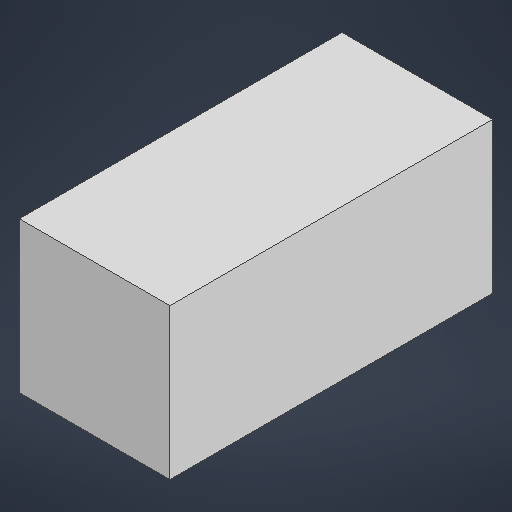
# Autodesk Inventor part: shootingstand
Saved by Autodesk Inventor 2026.2 (Build 302298000, 298)
## iProperties
Created: 2026-03-08
Part Number: shootingstand
Material: Generic
Document SubType Name: Modeling
Designer: danda
Density: 1 g/cm^3
Appearance: Default
Author: danda
Autodesk Inventor part; units mm, degrees
ref_plane "YZ Plane" through (0, 0, 0) normal (1, 0, 0) x (0, 1, 0)
ref_plane "XZ Plane" through (0, 0, 0) normal (0, 1, 0) x (-1, 0, 0)
ref_plane "XY Plane" through (0, 0, 0) normal (0, 0, 1) x (1, 0, 0)
sketch "Sketch1" plane through (0, 0, 0) normal (0, 0, 1) x (1, 0, 0)
  line L0 (11.218, 88.3381) -> (81.218, 88.3381)
  line L1 (81.218, 88.3381) -> (81.218, 18.3381)
  line L2 (81.218, 18.3381) -> (11.218, 18.3381)
  line L3 (11.218, 18.3381) -> (11.218, 88.3381)
  line L4 (11.218, 88.3381) -> (81.218, 18.3381) construction
  line L5 (81.218, 88.3381) -> (11.218, 18.3381) construction
  point P0 (0, 0)
  point P1 (46.218, 53.3381)
  dimension "d0" = 70
  dimension "d1" = 70
  constraints: 12 end point, 2 midpoint, 2 parallel, 1 horizontal, 1 perpendicular
  measures "d0" distance of L1.end L2.end
  measures "d1" distance of L0.end L1.end
extrude "Extrusion1" add sketch "Sketch1" along normal blind 150
body "Solid1"
